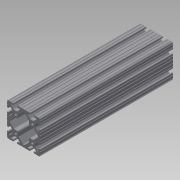
# Autodesk Inventor part: 3030
Saved by Autodesk Inventor 2013 (Build 170138000, 138)
## iProperties
Created: 2014-04-23
Part Number: 3030
Material: Generic
Document SubType Name: Modeling
Density: 1 g/cm^3
Vendor: 80/20 Inc.
Engineer: Ross Bowman
Designer: Ross Bowman
Catalog Web Link: 8020.net
Company: 80/20 Inc.
Author: Ross Bowman
Keywords: 80/20 , 8020 , T-Slot , Extrusion
Material: 6105-T5 Aluminum
Autodesk Inventor part; units mm, degrees
ref_plane "YZ Plane" through (0, 0, 0) normal (1, 0, 0) x (0, 1, 0)
ref_plane "XZ Plane" through (0, 0, 0) normal (0, 1, 0) x (-1, 0, 0)
ref_plane "XY Plane" through (0, 0, 0) normal (0, 0, 1) x (1, 0, 0)
sketch "Sketch1" plane through (0, 0, 0) normal (0, 0, 1) x (1, 0, 0)
  circle A0 centre (19.05, 19.05) radius 3.3274
  circle A1 centre (19.05, -19.05) radius 3.3274
  circle A2 centre (-19.05, -19.05) radius 3.3274
  circle A3 centre (-19.05, 19.05) radius 3.3274
  line L0 (2.0515, -32.1555) -> (11.3637, -22.8433)
  arc A4 (0, -33.011) -> (2.0515, -32.1555) centre (-0.0139, -30.09) ccw
  arc A5 (-2.0515, -32.1555) -> (0, -33.011) centre (0.0139, -30.09) ccw
  line L1 (-11.3637, -22.8433) -> (-2.0515, -32.1555)
  arc A6 (-12.2936, -20.5983) -> (-11.3637, -22.8433) centre (-9.1186, -20.5983) ccw
  line L2 (-12.2936, -15.4686) -> (-12.2936, -20.5983)
  arc A7 (-12.2936, -15.4686) -> (-15.4686, -12.2936) centre (-15.4686, -15.4686) ccw
  line L3 (-20.769, -12.2936) -> (-15.4686, -12.2936)
  arc A8 (-23.0141, -11.3637) -> (-20.769, -12.2936) centre (-20.769, -9.1186) ccw
  line L4 (-31.9021, -2.4756) -> (-23.0141, -11.3637)
  arc A9 (-32.7287, 0) -> (-31.9021, -2.4756) centre (-29.8367, -0.4102) ccw
  arc A10 (-31.9021, 2.4756) -> (-32.7287, 0) centre (-29.8367, 0.4102) ccw
  line L5 (-23.0141, 11.3637) -> (-31.9021, 2.4756)
  arc A11 (-20.769, 12.2936) -> (-23.0141, 11.3637) centre (-20.769, 9.1186) ccw
  line L6 (-15.4686, 12.2936) -> (-20.769, 12.2936)
  arc A12 (-15.4686, 12.2936) -> (-12.2936, 15.4686) centre (-15.4686, 15.4686) ccw
  line L7 (-12.2936, 20.5983) -> (-12.2936, 15.4686)
  arc A13 (-11.3637, 22.8433) -> (-12.2936, 20.5983) centre (-9.1186, 20.5983) ccw
  line L8 (-2.0515, 32.1555) -> (-11.3637, 22.8433)
  arc A14 (0, 33.011) -> (-2.0515, 32.1555) centre (0.0139, 30.09) ccw
  arc A15 (2.0515, 32.1555) -> (0, 33.011) centre (-0.0139, 30.09) ccw
  line L9 (11.3637, 22.8433) -> (2.0515, 32.1555)
  arc A16 (12.2936, 20.5983) -> (11.3637, 22.8433) centre (9.1186, 20.5983) ccw
  line L10 (12.2936, 15.4686) -> (12.2936, 20.5983)
  arc A17 (12.2936, 15.4686) -> (15.4686, 12.2936) centre (15.4686, 15.4686) ccw
  line L11 (20.769, 12.2936) -> (15.4686, 12.2936)
  arc A18 (23.0141, 11.3637) -> (20.769, 12.2936) centre (20.769, 9.1186) ccw
  line L12 (31.9021, 2.4756) -> (23.0141, 11.3637)
  arc A19 (32.7287, 0) -> (31.9021, 2.4756) centre (29.8367, 0.4102) ccw
  arc A20 (31.9021, -2.4756) -> (32.7287, 0) centre (29.8367, -0.4102) ccw
  line L13 (23.0141, -11.3637) -> (31.9021, -2.4756)
  arc A21 (20.769, -12.2936) -> (23.0141, -11.3637) centre (20.769, -9.1186) ccw
  line L14 (15.4686, -12.2936) -> (20.769, -12.2936)
  arc A22 (15.4686, -12.2936) -> (12.2936, -15.4686) centre (15.4686, -15.4686) ccw
  line L15 (12.2936, -20.5983) -> (12.2936, -15.4686)
  arc A23 (11.3637, -22.8433) -> (12.2936, -20.5983) centre (9.1186, -20.5983) ccw
  arc A24 (-4.7773, 38.1) -> (-3.2537, 38.1) centre (-4.0155, 38.0824) ccw
  line L16 (-4.7773, 38.1) -> (-9.6053, 38.1)
  arc A25 (-11.1289, 38.1) -> (-9.6053, 38.1) centre (-10.3671, 38.0824) ccw
  line L17 (-11.1289, 38.1) -> (-13.4112, 38.1)
  arc A26 (-13.4112, 38.1) -> (-14.986, 36.5252) centre (-13.4112, 36.5252) ccw
  line L18 (-14.986, 36.5252) -> (-14.986, 35.6108)
  arc A27 (-14.986, 35.6108) -> (-13.4112, 34.036) centre (-13.4112, 35.6108) ccw
  line L19 (-13.4112, 34.036) -> (-9.652, 34.036)
  arc A28 (-8.763, 33.147) -> (-9.652, 34.036) centre (-9.652, 33.147) ccw
  line L20 (-8.763, 33.147) -> (-8.763, 32.4935)
  arc A29 (-9.0234, 31.8649) -> (-8.763, 32.4935) centre (-9.652, 32.4935) ccw
  line L21 (-9.0234, 31.8649) -> (-13.6907, 27.1976)
  arc A30 (-17.0493, 25.8064) -> (-13.6907, 27.1976) centre (-17.0493, 30.5562) ccw
  line L22 (-17.0493, 25.8064) -> (-21.0507, 25.8064)
  arc A31 (-24.4093, 27.1976) -> (-21.0507, 25.8064) centre (-21.0507, 30.5562) ccw
  line L23 (-24.4093, 27.1976) -> (-29.1002, 31.8885)
  arc A32 (-29.337, 32.7207) -> (-29.1002, 31.8885) centre (-28.4716, 32.5172) ccw
  line L24 (-29.337, 32.7207) -> (-29.337, 33.147)
  arc A33 (-28.448, 34.036) -> (-29.337, 33.147) centre (-28.448, 33.147) ccw
  line L25 (-28.448, 34.036) -> (-24.6888, 34.036)
  arc A34 (-24.6888, 34.036) -> (-23.114, 35.6108) centre (-24.6888, 35.6108) ccw
  line L26 (-23.114, 35.6108) -> (-23.114, 36.5252)
  arc A35 (-23.114, 36.5252) -> (-24.6888, 38.1) centre (-24.6888, 36.5252) ccw
  line L27 (-24.6888, 38.1) -> (-27.0772, 38.1)
  arc A36 (-28.6011, 38.1) -> (-27.0772, 38.1) centre (-27.8392, 38.0824) ccw
  line L28 (-28.6011, 38.1) -> (-33.4288, 38.1)
  arc A37 (-34.9527, 38.1) -> (-33.4288, 38.1) centre (-34.1907, 38.0824) ccw
  arc A38 (-34.9527, 38.1) -> (-37.0861, 37.1826) centre (-34.8521, 34.9266) ccw
  arc A39 (-37.0861, 37.1826) -> (-38.1, 34.8455) centre (-34.925, 34.8566) ccw
  arc A40 (-38.1, 33.373) -> (-38.1, 34.8455) centre (-37.9035, 34.1092) ccw
  line L29 (-38.1, 33.373) -> (-38.1, 28.5453)
  arc A41 (-38.1, 27.0238) -> (-38.1, 28.5453) centre (-37.9035, 27.7845) ccw
  line L30 (-38.1, 27.0238) -> (-38.1, 24.6302)
  arc A42 (-38.1, 24.6302) -> (-36.5252, 23.0554) centre (-36.5252, 24.6302) ccw
  line L31 (-36.5252, 23.0554) -> (-35.6108, 23.0554)
  arc A43 (-35.6108, 23.0554) -> (-34.036, 24.6302) centre (-35.6108, 24.6302) ccw
  line L32 (-34.036, 24.6302) -> (-34.036, 28.448)
  arc A44 (-33.147, 29.337) -> (-34.036, 28.448) centre (-33.147, 28.448) ccw
  line L33 (-33.147, 29.337) -> (-32.6643, 29.337)
  arc A45 (-32.0357, 29.0766) -> (-32.6643, 29.337) centre (-32.6643, 28.448) ccw
  line L34 (-32.0357, 29.0766) -> (-27.1976, 24.2385)
  arc A46 (-25.8064, 20.8799) -> (-27.1976, 24.2385) centre (-30.5562, 20.8799) ccw
  line L35 (-25.8064, 20.8799) -> (-25.8064, 17.2201)
  arc A47 (-27.1976, 13.8615) -> (-25.8064, 17.2201) centre (-30.5562, 17.2201) ccw
  line L36 (-27.1976, 13.8615) -> (-31.9489, 9.1101)
  arc A48 (-32.7869, 8.763) -> (-31.9489, 9.1101) centre (-32.7869, 9.9481) ccw
  line L37 (-32.7869, 8.763) -> (-33.0603, 8.763)
  arc A49 (-34.036, 9.7387) -> (-33.0603, 8.763) centre (-33.0603, 9.7387) ccw
  line L38 (-34.036, 9.7387) -> (-34.036, 13.4698)
  arc A50 (-34.036, 13.4698) -> (-35.6108, 15.0446) centre (-35.6108, 13.4698) ccw
  line L39 (-35.6108, 15.0446) -> (-36.5252, 15.0446)
  arc A51 (-36.5252, 15.0446) -> (-38.1, 13.4698) centre (-36.5252, 13.4698) ccw
  line L40 (-38.1, 13.4698) -> (-38.1, 11.075)
  arc A52 (-38.1, 9.552) -> (-38.1, 11.075) centre (-37.9035, 10.3135) ccw
  line L41 (-38.1, 9.552) -> (-38.1, 4.7238)
  arc A53 (-38.1, 3.2007) -> (-38.1, 4.7238) centre (-37.9035, 3.9622) ccw
  line L42 (-38.1, 3.2007) -> (-38.1, -3.2007)
  arc A54 (-38.1, -4.7238) -> (-38.1, -3.2007) centre (-37.9035, -3.9622) ccw
  line L43 (-38.1, -4.7238) -> (-38.1, -9.552)
  arc A55 (-38.1, -11.075) -> (-38.1, -9.552) centre (-37.9035, -10.3135) ccw
  line L44 (-38.1, -11.075) -> (-38.1, -13.4698)
  arc A56 (-38.1, -13.4698) -> (-36.5252, -15.0446) centre (-36.5252, -13.4698) ccw
  line L45 (-36.5252, -15.0446) -> (-35.6108, -15.0446)
  arc A57 (-35.6108, -15.0446) -> (-34.036, -13.4698) centre (-35.6108, -13.4698) ccw
  line L46 (-34.036, -13.4698) -> (-34.036, -9.7387)
  arc A58 (-33.0603, -8.763) -> (-34.036, -9.7387) centre (-33.0603, -9.7387) ccw
  line L47 (-33.0603, -8.763) -> (-32.7869, -8.763)
  arc A59 (-31.9489, -9.1101) -> (-32.7869, -8.763) centre (-32.7869, -9.9481) ccw
  line L48 (-31.9489, -9.1101) -> (-27.1976, -13.8615)
  arc A60 (-25.8064, -17.2201) -> (-27.1976, -13.8615) centre (-30.5562, -17.2201) ccw
  line L49 (-25.8064, -17.2201) -> (-25.8064, -20.8799)
  arc A61 (-27.1976, -24.2385) -> (-25.8064, -20.8799) centre (-30.5562, -20.8799) ccw
  line L50 (-27.1976, -24.2385) -> (-32.0357, -29.0766)
  arc A62 (-32.6643, -29.337) -> (-32.0357, -29.0766) centre (-32.6643, -28.448) ccw
  line L51 (-32.6643, -29.337) -> (-33.147, -29.337)
  arc A63 (-34.036, -28.448) -> (-33.147, -29.337) centre (-33.147, -28.448) ccw
  line L52 (-34.036, -28.448) -> (-34.036, -24.6302)
  arc A64 (-34.036, -24.6302) -> (-35.6108, -23.0554) centre (-35.6108, -24.6302) ccw
  line L53 (-35.6108, -23.0554) -> (-36.5252, -23.0554)
  arc A65 (-36.5252, -23.0554) -> (-38.1, -24.6302) centre (-36.5252, -24.6302) ccw
  line L54 (-38.1, -24.6302) -> (-38.1, -27.0238)
  arc A66 (-38.1, -28.5453) -> (-38.1, -27.0238) centre (-37.9035, -27.7845) ccw
  line L55 (-38.1, -28.5453) -> (-38.1, -33.373)
  arc A67 (-38.1, -34.8455) -> (-38.1, -33.373) centre (-37.9035, -34.1092) ccw
  arc A68 (-38.1, -34.8455) -> (-37.0861, -37.1826) centre (-34.925, -34.8566) ccw
  arc A69 (-37.0861, -37.1826) -> (-34.9527, -38.1) centre (-34.8521, -34.9266) ccw
  arc A70 (-33.4288, -38.1) -> (-34.9527, -38.1) centre (-34.1907, -38.0824) ccw
  line L56 (-33.4288, -38.1) -> (-28.6011, -38.1)
  arc A71 (-27.0772, -38.1) -> (-28.6011, -38.1) centre (-27.8392, -38.0824) ccw
  line L57 (-27.0772, -38.1) -> (-24.6888, -38.1)
  arc A72 (-24.6888, -38.1) -> (-23.114, -36.5252) centre (-24.6888, -36.5252) ccw
  line L58 (-23.114, -36.5252) -> (-23.114, -35.6108)
  arc A73 (-23.114, -35.6108) -> (-24.6888, -34.036) centre (-24.6888, -35.6108) ccw
  line L59 (-24.6888, -34.036) -> (-28.448, -34.036)
  arc A74 (-29.337, -33.147) -> (-28.448, -34.036) centre (-28.448, -33.147) ccw
  line L60 (-29.337, -33.147) -> (-29.337, -32.7207)
  arc A75 (-29.1002, -31.8885) -> (-29.337, -32.7207) centre (-28.4716, -32.5172) ccw
  line L61 (-29.1002, -31.8885) -> (-24.4093, -27.1976)
  arc A76 (-21.0507, -25.8064) -> (-24.4093, -27.1976) centre (-21.0507, -30.5562) ccw
  line L62 (-21.0507, -25.8064) -> (-17.0493, -25.8064)
  arc A77 (-13.6907, -27.1976) -> (-17.0493, -25.8064) centre (-17.0493, -30.5562) ccw
  line L63 (-13.6907, -27.1976) -> (-9.0234, -31.8649)
  arc A78 (-8.763, -32.4935) -> (-9.0234, -31.8649) centre (-9.652, -32.4935) ccw
  line L64 (-8.763, -32.4935) -> (-8.763, -33.147)
  arc A79 (-9.652, -34.036) -> (-8.763, -33.147) centre (-9.652, -33.147) ccw
  line L65 (-9.652, -34.036) -> (-13.4112, -34.036)
  arc A80 (-13.4112, -34.036) -> (-14.986, -35.6108) centre (-13.4112, -35.6108) ccw
  line L66 (-14.986, -35.6108) -> (-14.986, -36.5252)
  arc A81 (-14.986, -36.5252) -> (-13.4112, -38.1) centre (-13.4112, -36.5252) ccw
  line L67 (-13.4112, -38.1) -> (-11.1289, -38.1)
  arc A82 (-9.6053, -38.1) -> (-11.1289, -38.1) centre (-10.3671, -38.0824) ccw
  line L68 (-9.6053, -38.1) -> (-4.7773, -38.1)
  arc A83 (-3.2537, -38.1) -> (-4.7773, -38.1) centre (-4.0155, -38.0824) ccw
  line L69 (-3.2537, -38.1) -> (3.2537, -38.1)
  arc A84 (4.7773, -38.1) -> (3.2537, -38.1) centre (4.0155, -38.0824) ccw
  line L70 (4.7773, -38.1) -> (9.6053, -38.1)
  arc A85 (11.1289, -38.1) -> (9.6053, -38.1) centre (10.3671, -38.0824) ccw
  line L71 (11.1289, -38.1) -> (13.4112, -38.1)
  arc A86 (13.4112, -38.1) -> (14.986, -36.5252) centre (13.4112, -36.5252) ccw
  line L72 (14.986, -36.5252) -> (14.986, -35.6108)
  arc A87 (14.986, -35.6108) -> (13.4112, -34.036) centre (13.4112, -35.6108) ccw
  line L73 (13.4112, -34.036) -> (9.652, -34.036)
  arc A88 (8.763, -33.147) -> (9.652, -34.036) centre (9.652, -33.147) ccw
  line L74 (8.763, -33.147) -> (8.763, -32.4935)
  arc A89 (9.0234, -31.8649) -> (8.763, -32.4935) centre (9.652, -32.4935) ccw
  line L75 (9.0234, -31.8649) -> (13.6907, -27.1976)
  arc A90 (17.0493, -25.8064) -> (13.6907, -27.1976) centre (17.0493, -30.5562) ccw
  line L76 (17.0493, -25.8064) -> (21.0507, -25.8064)
  arc A91 (24.4093, -27.1976) -> (21.0507, -25.8064) centre (21.0507, -30.5562) ccw
  line L77 (24.4093, -27.1976) -> (29.1002, -31.8885)
  arc A92 (29.337, -32.7207) -> (29.1002, -31.8885) centre (28.4716, -32.5172) ccw
  line L78 (29.337, -32.7207) -> (29.337, -33.147)
  arc A93 (28.448, -34.036) -> (29.337, -33.147) centre (28.448, -33.147) ccw
  line L79 (28.448, -34.036) -> (24.6888, -34.036)
  arc A94 (24.6888, -34.036) -> (23.114, -35.6108) centre (24.6888, -35.6108) ccw
  line L80 (23.114, -35.6108) -> (23.114, -36.5252)
  arc A95 (23.114, -36.5252) -> (24.6888, -38.1) centre (24.6888, -36.5252) ccw
  line L81 (24.6888, -38.1) -> (27.0772, -38.1)
  arc A96 (28.6011, -38.1) -> (27.0772, -38.1) centre (27.8392, -38.0824) ccw
  line L82 (28.6011, -38.1) -> (33.4288, -38.1)
  arc A97 (34.9527, -38.1) -> (33.4288, -38.1) centre (34.1907, -38.0824) ccw
  arc A98 (34.9527, -38.1) -> (37.0861, -37.1826) centre (34.8521, -34.9266) ccw
  arc A99 (37.0861, -37.1826) -> (38.1, -34.8455) centre (34.925, -34.8566) ccw
  arc A100 (38.1, -33.373) -> (38.1, -34.8455) centre (37.9035, -34.1092) ccw
  line L83 (38.1, -33.373) -> (38.1, -28.5453)
  arc A101 (38.1, -27.0238) -> (38.1, -28.5453) centre (37.9035, -27.7845) ccw
  line L84 (38.1, -27.0238) -> (38.1, -24.6302)
  arc A102 (38.1, -24.6302) -> (36.5252, -23.0554) centre (36.5252, -24.6302) ccw
  line L85 (36.5252, -23.0554) -> (35.6108, -23.0554)
  arc A103 (35.6108, -23.0554) -> (34.036, -24.6302) centre (35.6108, -24.6302) ccw
  line L86 (34.036, -24.6302) -> (34.036, -28.448)
  arc A104 (33.147, -29.337) -> (34.036, -28.448) centre (33.147, -28.448) ccw
  line L87 (33.147, -29.337) -> (32.6643, -29.337)
  arc A105 (32.0357, -29.0766) -> (32.6643, -29.337) centre (32.6643, -28.448) ccw
  line L88 (32.0357, -29.0766) -> (27.1976, -24.2385)
  arc A106 (25.8064, -20.8799) -> (27.1976, -24.2385) centre (30.5562, -20.8799) ccw
  line L89 (25.8064, -20.8799) -> (25.8064, -17.2201)
  arc A107 (27.1976, -13.8615) -> (25.8064, -17.2201) centre (30.5562, -17.2201) ccw
  line L90 (27.1976, -13.8615) -> (31.9489, -9.1101)
  arc A108 (32.7869, -8.763) -> (31.9489, -9.1101) centre (32.7869, -9.9481) ccw
  line L91 (32.7869, -8.763) -> (33.0603, -8.763)
  arc A109 (34.036, -9.7387) -> (33.0603, -8.763) centre (33.0603, -9.7387) ccw
  line L92 (34.036, -9.7387) -> (34.036, -13.4698)
  arc A110 (34.036, -13.4698) -> (35.6108, -15.0446) centre (35.6108, -13.4698) ccw
  line L93 (35.6108, -15.0446) -> (36.5252, -15.0446)
  arc A111 (36.5252, -15.0446) -> (38.1, -13.4698) centre (36.5252, -13.4698) ccw
  line L94 (38.1, -13.4698) -> (38.1, -11.075)
  arc A112 (38.1, -9.552) -> (38.1, -11.075) centre (37.9035, -10.3135) ccw
  line L95 (38.1, -9.552) -> (38.1, -4.7238)
  arc A113 (38.1, -3.2007) -> (38.1, -4.7238) centre (37.9035, -3.9622) ccw
  line L96 (38.1, -3.2007) -> (38.1, 3.2007)
  arc A114 (38.1, 4.7238) -> (38.1, 3.2007) centre (37.9035, 3.9622) ccw
  line L97 (38.1, 4.7238) -> (38.1, 9.552)
  arc A115 (38.1, 11.075) -> (38.1, 9.552) centre (37.9035, 10.3135) ccw
  line L98 (38.1, 11.075) -> (38.1, 13.4698)
  arc A116 (38.1, 13.4698) -> (36.5252, 15.0446) centre (36.5252, 13.4698) ccw
  line L99 (36.5252, 15.0446) -> (35.6108, 15.0446)
  arc A117 (35.6108, 15.0446) -> (34.036, 13.4698) centre (35.6108, 13.4698) ccw
  line L100 (34.036, 13.4698) -> (34.036, 9.7387)
  arc A118 (33.0603, 8.763) -> (34.036, 9.7387) centre (33.0603, 9.7387) ccw
  line L101 (33.0603, 8.763) -> (32.7869, 8.763)
  arc A119 (31.9489, 9.1101) -> (32.7869, 8.763) centre (32.7869, 9.9481) ccw
  line L102 (31.9489, 9.1101) -> (27.1976, 13.8615)
  arc A120 (25.8064, 17.2201) -> (27.1976, 13.8615) centre (30.5562, 17.2201) ccw
  line L103 (25.8064, 17.2201) -> (25.8064, 20.8799)
  arc A121 (27.1976, 24.2385) -> (25.8064, 20.8799) centre (30.5562, 20.8799) ccw
  line L104 (27.1976, 24.2385) -> (32.0357, 29.0766)
  arc A122 (32.6643, 29.337) -> (32.0357, 29.0766) centre (32.6643, 28.448) ccw
  line L105 (32.6643, 29.337) -> (33.147, 29.337)
  arc A123 (34.036, 28.448) -> (33.147, 29.337) centre (33.147, 28.448) ccw
  line L106 (34.036, 28.448) -> (34.036, 24.6302)
  arc A124 (34.036, 24.6302) -> (35.6108, 23.0554) centre (35.6108, 24.6302) ccw
  line L107 (35.6108, 23.0554) -> (36.5252, 23.0554)
  arc A125 (36.5252, 23.0554) -> (38.1, 24.6302) centre (36.5252, 24.6302) ccw
  line L108 (38.1, 24.6302) -> (38.1, 27.0238)
  arc A126 (38.1, 28.5453) -> (38.1, 27.0238) centre (37.9035, 27.7845) ccw
  line L109 (38.1, 28.5453) -> (38.1, 33.373)
  arc A127 (38.1, 34.8455) -> (38.1, 33.373) centre (37.9035, 34.1092) ccw
  arc A128 (38.1, 34.8455) -> (37.0861, 37.1826) centre (34.925, 34.8566) ccw
  arc A129 (37.0861, 37.1826) -> (34.9527, 38.1) centre (34.8521, 34.9266) ccw
  arc A130 (33.4288, 38.1) -> (34.9527, 38.1) centre (34.1907, 38.0824) ccw
  line L110 (33.4288, 38.1) -> (28.6011, 38.1)
  arc A131 (27.0772, 38.1) -> (28.6011, 38.1) centre (27.8392, 38.0824) ccw
  line L111 (27.0772, 38.1) -> (24.6888, 38.1)
  arc A132 (24.6888, 38.1) -> (23.114, 36.5252) centre (24.6888, 36.5252) ccw
  line L112 (23.114, 36.5252) -> (23.114, 35.6108)
  arc A133 (23.114, 35.6108) -> (24.6888, 34.036) centre (24.6888, 35.6108) ccw
  line L113 (24.6888, 34.036) -> (28.448, 34.036)
  arc A134 (29.337, 33.147) -> (28.448, 34.036) centre (28.448, 33.147) ccw
  line L114 (29.337, 33.147) -> (29.337, 32.7207)
  arc A135 (29.1002, 31.8885) -> (29.337, 32.7207) centre (28.4716, 32.5172) ccw
  line L115 (29.1002, 31.8885) -> (24.4093, 27.1976)
  arc A136 (21.0507, 25.8064) -> (24.4093, 27.1976) centre (21.0507, 30.5562) ccw
  line L116 (21.0507, 25.8064) -> (17.0493, 25.8064)
  arc A137 (13.6907, 27.1976) -> (17.0493, 25.8064) centre (17.0493, 30.5562) ccw
  line L117 (13.6907, 27.1976) -> (9.0234, 31.8649)
  arc A138 (8.763, 32.4935) -> (9.0234, 31.8649) centre (9.652, 32.4935) ccw
  line L118 (8.763, 32.4935) -> (8.763, 33.147)
  arc A139 (9.652, 34.036) -> (8.763, 33.147) centre (9.652, 33.147) ccw
  line L119 (9.652, 34.036) -> (13.4112, 34.036)
  arc A140 (13.4112, 34.036) -> (14.986, 35.6108) centre (13.4112, 35.6108) ccw
  line L120 (14.986, 35.6108) -> (14.986, 36.5252)
  arc A141 (14.986, 36.5252) -> (13.4112, 38.1) centre (13.4112, 36.5252) ccw
  line L121 (13.4112, 38.1) -> (11.1289, 38.1)
  arc A142 (9.6053, 38.1) -> (11.1289, 38.1) centre (10.3671, 38.0824) ccw
  line L122 (9.6053, 38.1) -> (4.7773, 38.1)
  arc A143 (3.2537, 38.1) -> (4.7773, 38.1) centre (4.0155, 38.0824) ccw
  line L123 (3.2537, 38.1) -> (-3.2537, 38.1)
  point P0 (0, 0)
  constraints: 280 point on circle, 248 end point, 144 centre point
extrude "Extrusion1" add sketch "Sketch1" against normal blind 304.8
body "Solid1"
